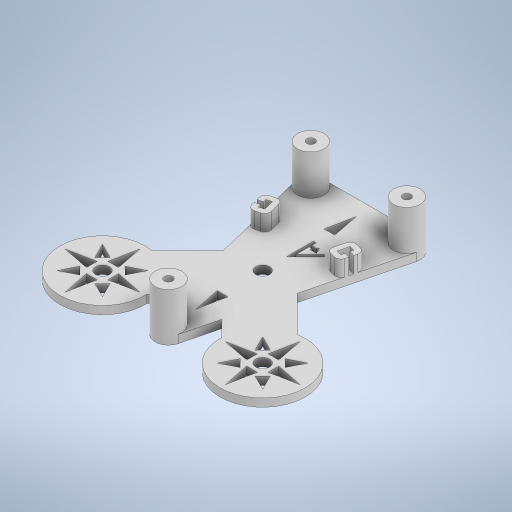
# Autodesk Inventor part: BaseLiDAR
Saved by Autodesk Inventor 2024.2 (Build 282272000, 272)
## iProperties
Created: 2024-07-17
Part Number: BaseLiDAR
Material: Generic
Document SubType Name: Modeling
Designer: jrcer
Density: 1 g/cm^3
Appearance: Default
Author: jrcer
Autodesk Inventor part; units mm, degrees
ref_plane "YZ Plane" through (0, 0, 0) normal (1, 0, 0) x (0, 1, 0)
ref_plane "XZ Plane" through (0, 0, 0) normal (0, 1, 0) x (-1, 0, 0)
ref_plane "XY Plane" through (0, 0, 0) normal (0, 0, 1) x (1, 0, 0)
sketch "Sketch1" plane through (0, 0, 0) normal (0, 1, 0) x (-1, 0, 0)
  circle A0 centre (0, 35.3) radius 1.55
  circle A1 centre (18, -36) radius 1.55
  circle A2 centre (-18, -36) radius 1.55
  circle A3 centre (0, 35.3) radius 5
  circle A4 centre (18, -36) radius 5
  circle A5 centre (-18, -36) radius 5
  point P0 (0, 0)
  dimension "d0" = 35.3
  dimension "d1" = 36
  dimension "d2" = 3.1
  dimension "d3" = 10
  dimension "d4" = 36
  dimension "d5" = 18
  constraints: 6 centre point, 4 equal radius, 3 coincident, 1 horizontal alignment, 1 vertical alignment
  measures "d0" distance of A0.centre point (0, 0)
  measures "d1" vertical distance of A2.centre point (0, 0)
  measures "d2" diameter of A0
  measures "d3" diameter of A3
  measures "d4" distance of A2.centre A1.centre
  measures "d5" horizontal distance of point (0, 0) A2.centre
extrude "Extrusion1" add sketch "Sketch1" along normal blind 15
sketch "Sketch2" plane through (0, 0, 35.3) normal (0, -1, 0) x (1, 0, 0)
  circle A0 centre (0, 0) radius 5 projected
  circle A1 centre (0, 0) radius 1.55 projected
  circle A2 centre (-18, -71.3) radius 1.55 projected
  circle A3 centre (-18, -71.3) radius 5 projected
  circle A4 centre (18, -71.3) radius 1.55 projected
  circle A5 centre (18, -71.3) radius 5 projected
  line L0 (-22.8479, -70.0761) -> (-4.8479, 1.2239)
  line L1 (22.8479, -70.0761) -> (4.8479, 1.2239)
  line L2 (-18, -76.3) -> (18, -76.3)
  circle A6 centre (0, -35.3) radius 2.6
  line L3 (-2, -60.3) -> (2, -60.3)
  line L4 (2, -60.3) -> (0, -70.3)
  line L5 (0, -70.3) -> (-2, -60.3)
  line L6 (0, -10.3) -> (-2, -20.3)
  line L7 (-2, -20.3) -> (2, -20.3)
  line L8 (2, -20.3) -> (0, -10.3)
  point P0 (0, -60.3)
  point P1 (0, -20.3)
  dimension "d8" = 5.2
  dimension "d73" = 4
  dimension "d74" = 10
  dimension "d76" = 15
  dimension "d77" = 25
  constraints: 18 end point, 6 point on circle, 5 tangent, 3 equal length, 3 horizontal, 3 vertical alignment, 2 midpoint, 1 centre point, 1 coincident
  measures "d8" diameter of A6
  measures "d73" distance of L3.start L3.end
  measures "d74" distance from line of L4.end L3
  measures "d76" distance from line of point (0, -35.3) L7
  measures "d77" distance from line of L3 point (0, -35.3)
extrude "Extrusion2" add sketch "Sketch2" along normal blind 3
sketch "Sketch3" plane through (0, 0, 35.3) normal (0, 1, 0) x (1, 0, 0)
  circle A0 centre (0, 35.3) radius 2.6 construction
  line L0 (0, 44.3) -> (1, 38.3)
  line L1 (1, 38.3) -> (-1, 38.3)
  line L2 (-3, 36.3) -> (-9, 35.3)
  line L3 (-1, 38.3) -> (0, 44.3)
  line L4 (-9, 35.3) -> (-3, 34.3)
  line L5 (-3, 34.3) -> (-3, 36.3)
  line L6 (2.6, 35.3) -> (-2.6, 35.3) construction
  line L7 (0, 37.9) -> (0, 32.7) construction
  line L8 (3, 36.3) -> (9, 35.3)
  line L9 (9, 35.3) -> (3, 34.3)
  line L10 (3, 34.3) -> (3, 36.3)
  line L11 (0, 26.3) -> (1, 32.3)
  line L12 (1, 32.3) -> (-1, 32.3)
  line L13 (-1, 32.3) -> (0, 26.3)
  line L14 (-1.8385, 37.1385) -> (1.8385, 33.4615) construction
  line L15 (1.8385, 37.1385) -> (-1.8385, 33.4615) construction
  line L16 (-4.2929, 39.5929) -> (-3, 36.8858)
  line L17 (-3, 36.8858) -> (-1.5858, 38.3)
  line L18 (-1.5858, 38.3) -> (-4.2929, 39.5929)
  line L19 (-1.8385, 37.1385) -> (-4.2929, 39.5929) construction
  line L20 (4.2929, 39.5929) -> (3, 36.8858)
  line L21 (3, 36.8858) -> (1.5858, 38.3)
  line L22 (1.5858, 38.3) -> (4.2929, 39.5929)
  line L23 (-4.2929, 31.0071) -> (-3, 33.7142)
  line L24 (-3, 33.7142) -> (-1.5858, 32.3)
  line L25 (-1.5858, 32.3) -> (-4.2929, 31.0071)
  line L26 (4.2929, 31.0071) -> (3, 33.7142)
  line L27 (1.5858, 32.3) -> (4.2929, 31.0071)
  line L28 (3, 33.7142) -> (1.5858, 32.3)
  circle A1 centre (-30, 5.3) radius 16
  circle A2 centre (0, 35.3) radius 29.9 construction
  line L29 (0, 35.3) -> (-30, 5.3) construction
  line L30 (0, 35.3) -> (-30, 35.3) construction
  circle A3 centre (-30, 5.3) radius 2.6 construction
  line L31 (-28, 9.3) -> (-32, 9.3)
  line L32 (-32, 9.3) -> (-30, 19.3)
  line L33 (-30, 19.3) -> (-28, 9.3)
  line L34 (-27.4, 5.3) -> (-32.6, 5.3) construction
  line L35 (-30, 2.7) -> (-30, 7.9) construction
  line L36 (-30, 5.3) -> (-30, 35.3) construction
  line L37 (-26, 3.3) -> (-26, 7.3)
  line L38 (-26, 7.3) -> (-16, 5.3)
  line L39 (-16, 5.3) -> (-26, 3.3)
  line L40 (-24.3431, 8.1284) -> (-27.1716, 10.9569)
  line L41 (-27.1716, 10.9569) -> (-21.5147, 13.7853)
  line L42 (-24.3431, 8.1284) -> (-21.5147, 13.7853)
  circle A4 centre (-30, 5.3) radius 2.6
  line L43 (-24.3431, 2.4716) -> (-27.1716, -0.3569)
  line L44 (-27.1716, -0.3569) -> (-21.5147, -3.1853)
  line L45 (-24.3431, 2.4716) -> (-21.5147, -3.1853)
  line L46 (-35.6569, 8.1284) -> (-32.8284, 10.9569)
  line L47 (-32.8284, 10.9569) -> (-38.4853, 13.7853)
  line L48 (-35.6569, 8.1284) -> (-38.4853, 13.7853)
  line L49 (-35.6569, 2.4716) -> (-38.4853, -3.1853)
  line L50 (-32.8284, -0.3569) -> (-38.4853, -3.1853)
  line L51 (-35.6569, 2.4716) -> (-32.8284, -0.3569)
  line L52 (-34, 3.3) -> (-34, 7.3)
  line L53 (-34, 7.3) -> (-44, 5.3)
  line L54 (-44, 5.3) -> (-34, 3.3)
  line L55 (-28, 1.3) -> (-32, 1.3)
  line L56 (-32, 1.3) -> (-30, -8.7)
  line L57 (-30, -8.7) -> (-28, 1.3)
  circle A5 centre (0, 0) radius 5 projected
  line L58 (-4.8479, -1.2239) -> (-22.8479, 70.0761) projected
  line L59 (-13.8479, 34.4261) -> (-27.2178, 21.0562)
  line L60 (-8.1467, 11.8431) -> (-14.0143, 5.9755)
  point P0 (0, 38.3)
  point P1 (0, 32.3)
  point P2 (-2.2929, 37.5929)
  point P3 (-25.7574, 9.5426)
  point P4 (0, 35.3)
  dimension "d11" = 3
  dimension "d12" = 6
  dimension "d13" = 2
  dimension "d14" = 3
  dimension "d15" = 45
  dimension "d16" = 45
  dimension "d17" = 3
  dimension "d41" = 59.8
  dimension "d49" = 30
  dimension "d50" = 45
  dimension "d51" = 32
  dimension "d52" = 5.2
  dimension "d53" = 4
  dimension "d54" = 10
  dimension "d55" = 4
  dimension "d56" = 4
  dimension "d57" = 4
  dimension "d58" = 6
  dimension "d59" = 6
  dimension "d70" = 20
  dimension "d71" = 45
  constraints: 120 end point, 31 symmetric about line, 14 midpoint, 9 equal length, 6 point on circle, 5 horizontal, 5 vertical alignment, 4 centre point, 4 horizontal alignment, 4 point on line, 4 vertical, 3 coincident, 2 perpendicular, 1 collinear, 1 concentric, 1 parallel, 10 other
  measures "d11" distance from line of point (0, 35.3) L1
  measures "d12" distance of point (0, 38.3) L0.start
  measures "d13" distance of L0.end L1.end
  measures "d14" distance between parallel lines of L7 L5
  measures "d15" angle of L6 L14
  measures "d16" angle of L6 L15
  measures "d17" distance of L17.end L16.start
  measures "d41" diameter of A2
  measures "d49" distance of L29.start L30.end
  measures "d50" angle of L30 L29
  measures "d51" diameter of A1
  measures "d52" diameter of A3
  measures "d53" distance of L31.start L31.end
  measures "d54" distance from line of L32.end L31
  measures "d55" distance from line of L31 L36.start
  measures "d56" distance from line of L29.end L37
  measures "d57" distance of L40.start L40.end
  measures "d58" distance from line of L41.end L40
  measures "d59" distance from line of L29.end L40
  measures "d70" distance between parallel lines of L59 L60
  measures "d71" angle of L30 L59
extrude "Extrusion3" add sketch "Sketch3" against normal blind 3 contours A1 | A1 L59 L58 L60
sketch "Sketch4" plane through (0, 0, 35.3) normal (0, 1, 0) x (1, 0, 0)
  line L0 (0, 54.3) -> (0, 44.3)
  line L1 (0, 44.3) -> (7.0711, 51.3711)
  line L2 (6.364, 52.0782) -> (1, 46.7142)
  line L3 (1, 46.7142) -> (1, 54.3)
  line L4 (0, 54.3) -> (1, 54.3)
  line L5 (6.364, 52.0782) -> (7.0711, 51.3711)
  arc A0 (4.5355, 50.2497) -> (1, 51.7142) centre (1, 46.7142) ccw
  arc A1 (5.2426, 50.9569) -> (1, 52.7142) centre (1, 46.7142) ccw
  arc A2 (4.8891, 50.6033) -> (1, 52.2142) centre (1, 46.7142) ccw construction
  line L6 (2.0015, 51.0433) -> (3.3256, 53.1638)
  line L7 (3.3256, 53.1638) -> (4.5, 50.9569)
  line L8 (4.5, 50.9569) -> (2.0015, 51.0433)
  point P0 (0, 35.3)
  point P1 (3.2757, 51.7213)
  point P2 (2.8602, 52.4186)
  point P3 (2.3112, 51.5392)
  dimension "d21" = 45
  dimension "d22" = 10
  dimension "d23" = 9
  dimension "d24" = 1
  dimension "d25" = 5
  dimension "d26" = 6
  dimension "d27" = 5.5
  dimension "d72" = 2.5
  constraints: 18 end point, 8 point on circle, 6 point on line, 3 centre point, 3 coincident, 1 equal length, 1 horizontal, 1 horizontal alignment, 1 perpendicular, 1 vertical, 1 vertical alignment, 8 other
  measures "d21" angle of L0 L1
  measures "d22" distance of L0.start L0.end
  measures "d23" distance of L0.end point (0, 35.3)
  measures "d24" distance between parallel lines of L1 L2
  measures "d25" radius of A0
  measures "d26" radius of A1
  measures "d27" radius of A2
  measures "d72" distance of L6.end L7.end
extrude "Extrusion4" cut sketch "Sketch4" against normal blind 1.5 contours L4 L3 L2 L5 L1 L0 | A1 L6 A0 L3 | L6 L7 A1 | A1 L7 L8 A0 L6 | A0 L8 L6
sketch "Sketch5" plane through (0, 0, 35.3) normal (0, 1, 0) x (1, 0, 0)
  circle A0 centre (18, 71.3) radius 1.55 construction
  line L0 (22.8479, 70.0761) -> (4.8479, -1.2239) construction
  line L1 (13.084, 55.9126) -> (18.9015, 54.444)
  line L2 (18.9015, 54.444) -> (16.9433, 46.6874)
  line L3 (16.9433, 46.6874) -> (11.1258, 48.156)
  line L4 (11.1258, 48.156) -> (13.084, 55.9126)
  line L5 (11.1258, 48.156) -> (18.9015, 54.444) construction
  line L6 (16.9433, 46.6874) -> (13.084, 55.9126) construction
  line L7 (13.5545, 49.6056) -> (15.4937, 49.1161)
  line L8 (15.4937, 49.1161) -> (16.4728, 52.9944)
  line L9 (16.4728, 52.9944) -> (14.5336, 53.4839)
  line L10 (14.5336, 53.4839) -> (13.5545, 49.6056)
  line L11 (17.7388, 49.8385) -> (15.7997, 50.328)
  line L12 (18.106, 51.2929) -> (16.1668, 51.7824)
  line L13 (0, 44.3) -> (0, 54.3) construction
  line L14 (-13.084, 55.9126) -> (-18.9015, 54.444)
  line L15 (-18.9015, 54.444) -> (-16.9433, 46.6874)
  line L16 (-16.9433, 46.6874) -> (-11.1258, 48.156)
  line L17 (-11.1258, 48.156) -> (-13.084, 55.9126)
  line L18 (-11.1258, 48.156) -> (-18.9015, 54.444) construction
  line L19 (-16.9433, 46.6874) -> (-13.084, 55.9126) construction
  line L20 (-13.5545, 49.6056) -> (-15.4937, 49.1161)
  line L21 (-15.4937, 49.1161) -> (-16.4728, 52.9944)
  line L22 (-16.4728, 52.9944) -> (-14.5336, 53.4839)
  line L23 (-14.5336, 53.4839) -> (-13.5545, 49.6056)
  line L24 (-17.7388, 49.8385) -> (-15.7997, 50.328)
  line L25 (-18.106, 51.2929) -> (-16.1668, 51.7824)
  point P0 (0, 35.3)
  point P1 (15.0137, 51.3)
  point P2 (15.0137, 51.3)
  point P3 (-15.0137, 51.3)
  point P4 (-15.0137, 51.3)
  dimension "d31" = 8
  dimension "d32" = 20
  dimension "d33" = 6
  dimension "d34" = 2
  dimension "d35" = 3.25
  dimension "d36" = 3.25
  constraints: 48 end point, 14 symmetric about line, 9 point on line, 4 parallel, 4 perpendicular, 2 midpoint, 1 collinear, 3 other
  measures "d31" distance of L3.end L1.start
  measures "d32" vertical distance of A0.centre point (15.014, 51.3)
  measures "d33" distance of L1.start L1.end
  measures "d34" distance between parallel lines of L3 L7
  measures "d35" distance between parallel lines of L3 L11
  measures "d36" distance between parallel lines of L1 L12
extrude "Extrusion5" add sketch "Sketch5" along normal blind 6 contours L1 L2 L12 L8 L9 L10 L7 L11 L3 L4 | L17 L16 L15 L24 L21 L20 L23 L22 L25 L14
fillet "Fillet1" radius 2 8 edges at (-11.1258, 3, -12.856) (-16.9433, 3, -11.3874) (-13.084, 3, -20.6126) (16.9433, 3, -11.3874) (11.1258, 3, -12.856) (18.9015, 3, -19.144) (-18.9015, 3, -19.144) (13.084, 3, -20.6126)
mirror "Mirror1" about plane through (0, 0, 0) normal (1, 0, 0) of "Extrusion3"
equation "\"d5\" = 0.5 * d4"
equation "\"d14\" = d11"
equation "\"d36\" = d35"
body "Solid1"
